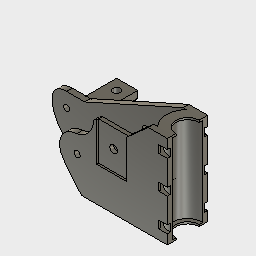
LeftZBrace v11 (Autodesk Fusion 360 design; units mm, degrees)
Autodesk Fusion 360 part; units mm, degrees
box "BoxPrimitive1" add length 21 width 78 height 48 placed x (0, 1, 0) y (-1, 0, 0) z (0, 0, 1) at (0, 0, 0) makes body 1
cylinder "CylinderPrimitive1" cut diameter 12 height -1 placed x (1, 0, 0) y (0, 1, 0) z (0, 0, 1) at (0, 10.5, 48) bodies 1
cylinder "CylinderPrimitive2" cut diameter 16 height -46 placed x (1, 0, 0) y (0, 1, 0) z (0, 0, 1) at (0, 10.5, 47) bodies 1
sketch "Sketch4" plane through (0, 0, 1) normal (0, 0, 1) x (-1, 0, 0)
  line L0 (0, -2.5) -> (0, -18.5)
  arc A0 (0, -18.5) -> (0, -2.5) centre (0, -10.5) ccw
  arc A1 (0, -16.5) -> (0, -4.5) centre (0, -10.5) ccw
extrude "Extrude1" cut sketch "Sketch4" against normal blind 1 contours L0 A1 bodies 1
sketch "Sketch5" plane through (0, 0, 0) normal (1, 0, 0) x (0, 1, 0)
  line L0 (4.5, 0) -> (4.5, 1)
  line L1 (4.5, 1) -> (2.5, 1)
  line L2 (2.5, 1) -> (2.5, 47)
  line L3 (2.5, 47) -> (4.5, 47)
  line L4 (4.5, 47) -> (4.5, 48)
  line L5 (4.5, 48) -> (0, 48)
  line L6 (0, 48) -> (0, 0)
  line L7 (0, 0) -> (4.5, 0)
  line L8 (0, 48) -> (0, 0)
  line L9 (0, 43) -> (1.5, 43)
  line L10 (1.5, 43) -> (1.5, 39)
  line L11 (1.5, 39) -> (0, 39)
  line L12 (0, 26) -> (1.5, 26)
  line L13 (1.5, 26) -> (1.5, 22)
  line L14 (1.5, 26) -> (5.5, 26) construction
  line L15 (1.5, 22) -> (0, 22)
  line L16 (0, 9) -> (1.5, 9)
  line L17 (1.5, 9) -> (1.5, 5)
  line L18 (1.5, 9) -> (5.5, 9) construction
  line L19 (1.5, 5) -> (0, 5)
  dimension "d12" = 5
  dimension "d13" = 4
  dimension "d14" = 1.5
  dimension "d15" = 1.5
  dimension "d16" = 90
  dimension "d17" = 4
  dimension "d18" = 180
  dimension "d19" = 1.5
  dimension "d20" = 1.5
  dimension "d21" = 90
  dimension "d22" = 4
  dimension "d23" = 180
  dimension "d24" = 1.5
  dimension "d25" = 13
  dimension "d26" = 13
  constraint coincident L6
  constraint perpendicular L6 L9
  constraint perpendicular L9 L10
  constraint coincident L8
  constraint horizontal L11
  constraint horizontal L14
  constraint horizontal L18
  measures "d12" distance of L5 L9
  measures "d13" distance of L9 L11
  measures "d16" angle of L13 L14
  measures "d18" angle of L14 L15
  measures "d21" angle of L17 L18
  measures "d23" angle of L18 L19
  measures "d25" distance of L11 L12
  measures "d26" distance of L15 L16
revolve "Revolve1" cut sketch "Sketch5" angle 180 about axis through (0, 10.5, 93) along (0, 0, -1) contours L6 L8 L16 L17 L19 | L6 L8 L12 L13 L15 | L6 L8 L9 L10 L11 bodies 1
sketch "Sketch6" plane through (0, 21, 0) normal (0, 1, 0) x (-1, 0, 0)
  line L0 (0, 48) -> (0, 43)
  line L1 (0, 43) -> (0, 39)
  line L2 (0, 39) -> (0, 26)
  line L3 (0, 26) -> (0, 22)
  line L4 (0, 22) -> (0, 9)
  line L5 (0, 9) -> (0, 5)
  line L6 (0, 5) -> (0, 0)
  line L7 (0, 0) -> (78, 0)
  line L8 (78, 0) -> (78, 48)
  line L9 (78, 48) -> (0, 48)
  line L10 (0, 43) -> (4.5, 43)
  line L11 (4.5, 43) -> (4.5, 39)
  line L12 (4.5, 39) -> (0, 39)
  line L13 (0, 26) -> (4.5, 26)
  line L14 (4.5, 26) -> (4.5, 22)
  line L15 (4.5, 22) -> (0, 22)
  line L16 (0, 9) -> (4.5, 9)
  line L17 (4.5, 9) -> (4.5, 5)
  line L18 (4.5, 5) -> (0, 5)
  dimension "d28" = 4.5
  constraint perpendicular L1 L10
  constraint perpendicular L10 L11
  constraint perpendicular L11 L13
  constraint perpendicular L13 L14
  constraint perpendicular L5 L16
  constraint perpendicular L16 L17
extrude "Extrude2" cut sketch "Sketch6" against normal blind 1 contours L1 L10 L11 L12 | L3 L13 L14 L15 | L5 L16 L17 L18 bodies 1
sketch "Sketch7" plane through (0, 0, 0) normal (0, -1, 0) x (1, 0, 0)
  line L0 (-78, 48) -> (-78, 0)
  line L1 (-78, 0) -> (0, 0)
  line L2 (0, 0) -> (0, 5)
  line L3 (0, 5) -> (0, 9)
  line L4 (0, 9) -> (0, 22)
  line L5 (0, 22) -> (0, 26)
  line L6 (0, 26) -> (0, 39)
  line L7 (0, 39) -> (0, 43)
  line L8 (0, 43) -> (0, 48)
  line L9 (0, 48) -> (-78, 48)
  line L10 (-4.5, 39) -> (0, 39)
  line L11 (-4.4721, 39) -> (-4.4721, 43)
  line L12 (-10.5, 43) -> (0, 43)
  line L13 (0, 43) -> (0, 39)
  line L14 (-10.5, 39) -> (0, 39)
  line L15 (-4.4721, 22) -> (-4.4721, 26)
  line L16 (-10.5, 26) -> (0, 26)
  line L17 (0, 26) -> (0, 22)
  line L18 (-10.5, 22) -> (0, 22)
  line L19 (-4.4721, 5) -> (-4.4721, 9)
  line L20 (-10.5, 9) -> (0, 9)
  line L21 (0, 9) -> (0, 5)
  line L22 (-10.5, 5) -> (0, 5)
  line L23 (-36.8, 37.98) -> (-36.8, 18)
  line L24 (-36.8, 18) -> (-21.2, 18)
  line L25 (-21.2, 18) -> (-21.2, 37.98)
  line L26 (-21.2, 37.98) -> (-36.8, 37.98)
  line L27 (-10, 48) -> (-21.2, 37.98)
  arc A0 (-36.8, 37.98) -> (-38.494, 36.4732) centre (-36.8, 36.2743) ccw
  line L28 (-38.494, 36.4732) -> (-38.494, 36.9887)
  line L29 (0, 0) -> (-78, 0)
  arc A1 (-54.6849, 12.6263) -> (-44.5, 0) centre (1.6407, 47.6398) ccw
  circle A2 centre (-29.01, 28.25) radius 2
  circle A3 centre (-47, 17.5) radius 1.6
  arc A4 (-47.185, 26.5981) -> (-38.494, 36.9887) centre (-49.0509, 36.9887) ccw
  arc A5 (-47.185, 26.5981) -> (-54.6849, 12.6263) centre (-47, 17.5) ccw
  dimension "d37" = 15.6
  dimension "d38" = 19.98
  dimension "d39" = 18
  dimension "d40" = 21.2
  dimension "d43" = 10
  dimension "d44" = 4
  dimension "d45" = 3.2
  dimension "d46" = 9.73
  dimension "d47" = 7.81
  dimension "d48" = 10.25
  dimension "d49" = 47
  dimension "d50" = 17.5
  dimension "d52" = 44.5
  dimension "d53" = 7.5
  constraint perpendicular L14 L23
  constraint perpendicular L23 L24
  constraint perpendicular L24 L25
  constraint perpendicular L23 L26
  constraint coincident L9
  constraint tangent L26 A0
  constraint perpendicular L26 L28
  constraint coincident L1
  constraint tangent L28 A4
  constraint concentric A3 A5
  measures "d39" distance of L1 L24
  measures "d40" distance of L6 L25
  measures "d44" diameter of A2
  measures "d45" diameter of A3
  measures "d46" distance of L26
  measures "d47" distance of L25
  measures "d48" distance of L24
  measures "d49" distance of L4
  measures "d50" distance of L29
  measures "d53" distance of A3 A5
extrude "Extrude3" cut sketch "Sketch7" against normal blind 1 contours L7 L10 L11 L12 L13 L14 | L3 L19 L20 L21 L22 | L5 L15 L16 L17 L18 bodies 1
sketch "Sketch8" plane through (0, 0, 48) normal (0, 0, 1) x (-1, 0, 0)
  arc A0 (0, -16.5) -> (0, -4.5) centre (0, -10.5) ccw
  line L0 (0, -16.5) -> (0, -21)
  line L1 (0, -21) -> (78, -21)
  line L2 (78, -21) -> (78, 0)
  line L3 (78, 0) -> (0, 0)
  line L4 (0, 0) -> (0, -4.5)
  arc A1 (4.4721, -20) -> (4.4721, -1) centre (0, -10.5) ccw
  arc A2 (0, -19.5) -> (0, -1.5) centre (0, -10.5) ccw
  line L5 (8.0467, -3) -> (78, -3)
  line L6 (8.0467, -18) -> (78, -18)
  arc A3 (4.6851, -20.4524) -> (4.6851, -0.5476) centre (0, -10.5) ccw
  dimension "d33" = 0.5
  dimension "d34" = 3
  dimension "d35" = 3
  constraint coincident L2
  constraint perpendicular L2 L5
  constraint perpendicular L2 L6
  measures "d34" distance of L3 L5
  measures "d35" distance of L1 L6
extrude "Extrude4" cut sketch "Sketch8" against normal up to surface (48 mm away) contours L2 L5 L6 A3 bodies 1
extrude "Extrude5" cut sketch "Sketch7" against normal blind 1 contours L23 L24 L25 L26 | A2 bodies 1
extrude "Extrude6" cut sketch "Sketch7" against normal up to surface (3 mm away) contours L0 L1 L9 L26 L27 A0 L28 L29 A1 A4 A5 | A2 | A3 bodies 1
sketch "Sketch9" plane through (0, 21, 0) normal (0, 1, 0) x (-1, 0, 0)
  line L0 (4.5, 39) -> (0, 39)
  line L1 (0, 39) -> (0, 26)
  line L2 (0, 26) -> (4.5, 26)
  line L3 (4.5, 26) -> (4.5, 22)
  line L4 (4.5, 22) -> (0, 22)
  line L5 (0, 22) -> (0, 9)
  line L6 (0, 9) -> (4.5, 9)
  line L7 (4.5, 9) -> (4.5, 5)
  line L8 (4.5, 5) -> (0, 5)
  line L9 (0, 5) -> (0, 0)
  line L10 (0, 0) -> (78, 0)
  line L11 (78, 0) -> (78, 48)
  line L12 (78, 48) -> (0, 48)
  line L13 (0, 48) -> (0, 43)
  line L14 (0, 43) -> (4.5, 43)
  line L15 (4.5, 43) -> (4.5, 39)
  circle A0 centre (29.01, 28.25) radius 2
  circle A1 centre (22, 17.5) radius 1.6
  line L16 (78, 25) -> (61, 25)
  line L17 (61, 25) -> (9.8593, 48)
  circle A2 centre (70.5, 17.5) radius 1.6
  spline S0 degree 5 poles (70.5, 25) (71.2557, 25) (72.6666, 24.8966) (74.482, 24.4311) (76.3123, 23.2293) (77.6758, 20.969) (78.187, 18.203) (77.9237, 15.1721) (76.9805, 12.0456) (75.4552, 8.9236) (73.4305, 5.8602) (71.4595, 3.4739) (69.7994, 1.7224) (68.613, 0.5713) (68, 0) knots 0 0 0 0 0 0 0.1 0.2 0.3 0.4 0.5 0.6 0.7 0.8 0.9 1 1 1 1 1 1
  line L18 (66.4967, 25) -> (74.5033, 25)
  dimension "d55" = 3.2
  dimension "d56" = 22
  dimension "d57" = 17.5
  dimension "d58" = 25
  dimension "d59" = 17
  dimension "d60" = 3.2
  dimension "d61" = 7.5
  dimension "d62" = 17.5
  dimension "d63" = 9.5
  dimension "d64" = 10
  constraint coincident L11
  constraint perpendicular L11 L16
  constraint coincident L12
  constraint coincident L16
  constraint coincident L10
  constraint midpoint L18
  measures "d55" diameter of A1
  measures "d56" distance of L5
  measures "d57" distance of L10
  measures "d60" diameter of A2
  measures "d61" distance of L11
  measures "d62" distance of L10
extrude "Extrude7" cut sketch "Sketch9" against normal blind 3 contours L11 L12 L16 L17 L18 | L11 L16 S0 L18 | L10 L11 S0 | A0 | A1 | A2 bodies 1
sketch "Sketch10" plane through (0, 0, 25) normal (0, 0, 1) x (-1, 0, 0)
  line L0 (61, -21) -> (70.5, -21)
  line L1 (70.5, -21) -> (70.5, -18)
  line L2 (70.5, -18) -> (61, -18)
  line L3 (61, -18) -> (61, -21)
  line L4 (63.4, -21) -> (63.4, -37)
  line L5 (63.4, -37) -> (52.4, -37)
  line L6 (52.4, -37) -> (52.4, -21)
  line L7 (52.4, -21) -> (63.4, -21)
  circle A0 centre (57.9, -31.5) radius 1.9
  dimension "d67" = 7.1
  dimension "d68" = 2.4
  dimension "d69" = 11
  dimension "d70" = 16
  dimension "d71" = 3.8
  dimension "d72" = 5.5
  dimension "d73" = 5.5
  constraint coincident L0
  constraint perpendicular L0 L4
  constraint perpendicular L4 L5
  constraint perpendicular L0 L6
  constraint midpoint L5
  measures "d71" diameter of A0
  measures "d72" distance of L6
extrude "Extrude8" add sketch "Sketch10" against normal blind 3.5 separate body contours L0 L4 L5 L6 L7 makes body 2
ref_plane "WorkPlane1" through (-57.9, 29, 23.25) normal (-1, 0, 0) x (0, 1, 0)
sketch "Sketch11" plane through (-63.4, 0, 0) normal (-1, 0, 0) x (0, -1, 0)
  line L0 (-21, 25) -> (-37, 25)
  line L1 (-37, 25) -> (-37, 21.5)
  line L2 (-37, 21.5) -> (-21, 21.5)
  line L3 (-21, 21.5) -> (-21, 25)
  line L4 (-21, 25) -> (-21, 13.5)
  line L5 (-21, 25) -> (-9.5, 25) construction
  line L6 (-21, 13.5) -> (-37, 21.5)
  dimension "d76" = 90
  dimension "d77" = 11.5
  constraint horizontal L5
  measures "d76" angle of L4 L5
extrude "Extrude9" add sketch "Sketch11" against normal blind 2.5 separate body contours L2 L4 L6 makes body 3
mirror "Mirror1" about plane through (-57.9, 29, 23.25) normal (-1, 0, 0) of bodies 3 makes body 4
sketch "Sketch12" plane through (0, 18, 0) normal (0, -1, 0) x (1, 0, 0)
  spline S0 degree 5 poles (-78, 17.3085) (-77.9879, 16.8856) (-77.9131, 15.8587) (-77.6257, 14.1921) (-76.894, 11.8685) (-75.4552, 8.9236) (-73.4305, 5.8602) (-71.4595, 3.4739) (-69.7994, 1.7224) (-68.613, 0.5713) (-68, 0) knots 0.428364 0.428364 0.428364 0.428364 0.428364 0.428364 0.5 0.6 0.7 0.8 0.9 1 1 1 1 1 1
  line L0 (-68, 0) -> (-8.0467, 0)
  line L1 (-8.0467, 0) -> (-8.0467, 48)
  line L2 (-8.0467, 48) -> (-9.8593, 48)
  line L3 (-9.8593, 48) -> (-61, 25)
  line L4 (-61, 25) -> (-70.5, 25)
  spline S1 degree 5 poles (-70.5, 25) (-71.2557, 25) (-72.6666, 24.8966) (-74.482, 24.4311) (-76.3123, 23.2293) (-77.4195, 21.3939) (-77.8549, 19.7738) (-77.9785, 18.611) (-77.999, 17.9975) (-78, 17.9627) knots 0 0 0 0 0 0 0.1 0.2 0.3 0.4 0.406002 0.406002 0.406002 0.406002 0.406002 0.406002
  line L5 (-78, 17.9627) -> (-78, 17.3085)
  circle A0 centre (-70.5, 17.5) radius 1.6
  circle A1 centre (-22, 17.5) radius 1.6
  circle A2 centre (-29.01, 28.25) radius 2
  line L6 (0, 5) -> (0, 9)
  line L7 (-9, 9) -> (0, 9)
  line L8 (0, 9) -> (0, 5)
  line L9 (-9, 5) -> (0, 5)
  line L10 (-8.0467, 0) -> (-15.5467, 0) construction
  line L11 (-8.0467, 0) -> (-0.5467, 0) construction
  line L12 (-15.5467, 0) -> (-15.5467, 10) construction
  line L13 (-15.5467, 0) -> (-25.5467, 0) construction
  line L14 (-8.0467, 0) -> (-15.5467, 10)
  line L15 (-15.5467, 10) -> (-15.5467, 20)
  line L16 (-15.5467, 10) -> (-25.5467, 10) construction
  line L17 (-15.5467, 20) -> (-8.0467, 20)
  dimension "d81" = 180
  dimension "d82" = 7.5
  dimension "d83" = 90
  dimension "d84" = 10
  dimension "d85" = 12.5
  dimension "d86" = 10
  constraint horizontal L11
  constraint horizontal L13
  constraint parallel L12 L15
  constraint horizontal L16
  constraint coincident L1
  constraint perpendicular L1 L17
  measures "d81" angle of L10 L11
  measures "d83" angle of L12 L13
extrude "Extrude10" add sketch "Sketch12" along normal up to surface (15 mm away) separate body contours L1 L14 L15 L17 makes body 5
